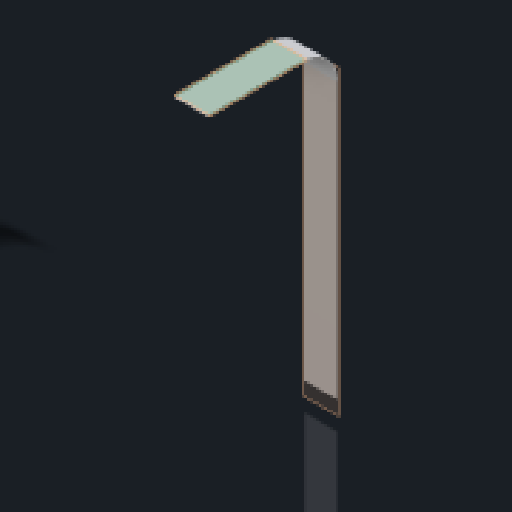
# Autodesk Inventor part: CARCASA_ALUM_9
Saved by Autodesk Inventor 2024.3 (Build 283343000, 343)
## iProperties
Created: 2024-05-15
Part Number: CARCASA_ALUM_9
Material: Generic
Document SubType Name: Sheet Metal
Designer: Niler
Density: 1 g/cm^3
Sheet Metal Rule: Default_mm
Appearance: Default
Author: Niler
Autodesk Inventor part; units mm, degrees
ref_plane "YZ Plane" through (0, 0, 0) normal (1, 0, 0) x (0, 1, 0)
ref_plane "XZ Plane" through (0, 0, 0) normal (0, 1, 0) x (-1, 0, 0)
ref_plane "XY Plane" through (0, 0, 0) normal (0, 0, 1) x (1, 0, 0)
ref_plane "Work Plane1" through (0, 0, 0) normal (0, 0, 1) x (1, 0, 0)
ref_plane "Work Plane2" through (0, 110, 380) normal (0, -1, 0) x (-1, 0, 0)
sketch "Sketch1" plane through (0, 0, 0) normal (0, 0, 1) x (1, 0, 0)
  line L0 (0, 0) -> (0, -840)
  line L1 (0, 0) -> (-100, 0)
  line L2 (-100, 0) -> (-100, -140)
  line L3 (-10, -140) -> (-100, -140)
  line L4 (-10, -140) -> (-10, -700)
  line L5 (-10, -700) -> (-100, -700)
  line L6 (-100, -700) -> (-100, -840)
  line L7 (0, -840) -> (-100, -840)
  line L8 (-100, -140) -> (-100, -700)
  line L9 (-100, -420) -> (0, -420)
extrude "Plate1" add sketch "Sketch1" against normal blind 1.5 contours L0 L9 L4 L3 L2 L1 | L9 L8 L3 L4
ref_plane "Work Plane3" through (0, 111.5, 380) normal (0, -1, 0) x (-1, 0, 0)
sketch "Sketch2" plane through (0, 111.5, 380) normal (0, -1, 0) x (-1, 0, 0)
  line L0 (0, 380) -> (100, 380)
  line L1 (100, 380) -> (100, -18.5)
  line L2 (100, -18.5) -> (0, -18.5)
  line L3 (0, -18.5) -> (0, 380)
  constraints: 8 end point
edge flange "Flange1" height 400 angle 90 thickness 1.5 bend radius 110 thickness toward (0, -1, 0) relief tear relief width 1.5 relief depth 0.75 edges at (-50, 0, 0) wall of the first edge with corners at (0, 111.5, 0) (-100, 111.5, 0) (-100, 111.5, 398.5) (0, 111.5, 398.5)
bend "Bend1"
corner "Corner1"
equation "\"d0\" = Thickness"
equation "\"d2\" = BendReliefWidth"
equation "\"d3\" = BendReliefDepth"
equation "\"d4\" = MinimumRemnant"
equation "\"d5\" = TransitionRadius"
equation "\"d9\" = CornerReliefSize"
equation "\"d10\" = GapSize"
equation "\"d11\" = JacobiRadiusSize"
equation "\"BendRadius\" = Thickness"
equation "\"BendReliefWidth\" = Thickness"
equation "\"BendReliefDepth\" = 0.5 * Thickness"
equation "\"CornerReliefSize\" = 4 * Thickness"
equation "\"MinimumRemnant\" = 2 * Thickness"
equation "\"TransitionRadius\" = BendRadius"
equation "\"JacobiRadiusSize\" = BendRadius"
equation "\"GapSize\" = Thickness"
equation "\"Thickness\" = 1.5"
body "Solid1"
